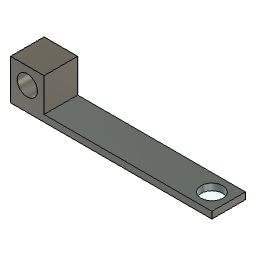
Ender 6 Extruder Bowden Tube Mount (Autodesk Fusion 360 design; units mm, degrees)
Autodesk Fusion 360 part; units mm, degrees
sketch "Sketch1" plane through (0, 0, 0) normal (0, 0, 1) x (1, 0, 0)
  line L0 (0, 0) -> (60, 0)
  line L1 (60, 0) -> (60, 10)
  line L2 (60, 10) -> (0, 10)
  line L3 (0, 10) -> (0, 0)
  dimension "d1" = 60
  dimension "d2" = 10
  constraint horizontal L0
  constraint vertical L1
  constraint horizontal L2
  constraint vertical L3
  constraint coincident L0.start L3.end
  measures "d1" distance of L0.start L0.end
  measures "d2" distance of L0.start L2.end
extrude "Extrude1" add sketch "Sketch1" along normal blind 2
hole "Hole1" at (55, 5, 2) direction (0, 0, -1) diameter 3.4 depth 8.6 tip angle 180 counterbore diameter 6.5 counterbore depth 3
sketch "Sketch2" plane through (0, 0, 0) normal (-1, 0, 0) x (0, -1, 0)
  line L0 (-10, 0) -> (0, 0)
  line L1 (0, 0) -> (0, 2)
  line L2 (0, 2) -> (-10, 2)
  line L3 (-10, 2) -> (-10, 0)
  line L4 (0, 2) -> (-10, 2)
  line L5 (-10, 2) -> (-10, 12)
  line L6 (-10, 12) -> (0, 12)
  line L7 (0, 12) -> (0, 2)
  dimension "d12" = 10
  dimension "d13" = 10
  constraint horizontal L4
  constraint vertical L5
  constraint horizontal L6
  constraint vertical L7
  constraint coincident L1.end L2.start
  measures "d12" distance of L1.end L2.end
  measures "d13" distance of L1.end L6.end
extrude "Extrude2" add sketch "Sketch2" against normal blind 10 contours L2 L4 L5 L6 L7
hole "Hole2" at (5, 0, 7) direction (0, 1, 0) diameter 6 depth 12 tip angle 180
sketch "Sketch3" plane through (0, 0, 2) normal (0, 0, 1) x (-1, 0, 0)
  line L0 (-10, -10) -> (-10, 0)
  line L1 (-10, 0) -> (-60, 0)
  line L2 (-60, 0) -> (-60, -10)
  line L3 (-60, -10) -> (-10, -10)
  circle A0 centre (-55, -5) radius 3.25
